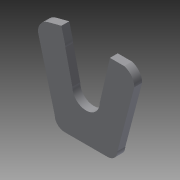
# Autodesk Inventor part: 4-2
Saved by Autodesk Inventor 2015 SP2 (Build 190223200, 223)
## iProperties
Created: 2015-09-16
Part Number: 4-2
Material: Generic
Document SubType Name: Modeling
Designer: Brandon
Density: 1 g/cm^3
Appearance: Default
Author: Brandon
Autodesk Inventor part; units mm, degrees
ref_plane "YZ Plane" through (0, 0, 0) normal (1, 0, 0) x (0, 1, 0)
ref_plane "XZ Plane" through (0, 0, 0) normal (0, 1, 0) x (-1, 0, 0)
ref_plane "XY Plane" through (0, 0, 0) normal (0, 0, 1) x (1, 0, 0)
sketch "Sketch1" plane through (0, 0, 0) normal (0, 0, 1) x (1, 0, 0)
  arc A0 (-22.225, 0) -> (22.225, 0) centre (0, 0) ccw
  arc A1 (34.925, -69.85) -> (50.8, -53.975) centre (34.925, -53.975) ccw
  arc A2 (-50.8, -53.975) -> (-34.925, -69.85) centre (-34.925, -53.975) ccw
  line L0 (-34.925, -69.85) -> (34.925, -69.85)
  line L1 (-50.8, -53.975) -> (-78.105, 49.53)
  line L2 (50.8, -53.975) -> (78.105, 49.53)
  line L3 (-33.655, 49.53) -> (-22.225, 0)
  line L4 (33.655, 49.53) -> (22.225, 0)
  line L5 (-61.5491, 71.0198) -> (-39.9288, 76.7156)
  line L6 (-39.9288, 76.7156) -> (-34.3567, 55.0708)
  line L7 (61.5491, 71.0198) -> (38.6142, 71.0198)
  line L8 (38.6142, 71.0198) -> (32.2206, 43.3143)
  arc A3 (-33.655, 49.53) -> (-34.3567, 55.0708) centre (-55.88, 49.53) ccw
  arc A4 (-61.5347, 71.0236) -> (-75.2129, 38.5669) centre (-55.88, 49.53) ccw
  arc A5 (75.2129, 38.5669) -> (50.2109, 71.0198) centre (55.88, 49.53) ccw
  arc A6 (35.9025, 59.269) -> (33.655, 49.53) centre (55.88, 49.53) ccw
  dimension "d1" = 31.75
  dimension "d5" = 31.75
  dimension "d8" = 34.925
  dimension "d11" = 69.85
  dimension "d15" = 119.38
  dimension "d16" = 55.88
  constraints: 18 end point, 18 point on circle, 7 centre point, 6 point on line, 2 horizontal, 1 coincident, 1 tangent
  measures "d1" diameter of A1
  measures "d5" diameter of A2
  measures "d8" horizontal distance of A1.centre point (0, 0)
  measures "d11" distance from line of L0 point (0, 0)
  measures "d15" distance from line of L0 A5.centre
  measures "d16" horizontal distance of point (0, 0) A5.centre
extrude "Extrusion1" add sketch "Sketch1" along normal blind 12.7 contours A0 L4 L8 L7 A5 L2 A1 L0 A2 L1 A4 L5 L6 A3 L3
body "Solid1"
